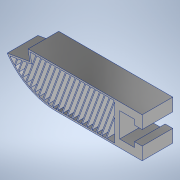
# Autodesk Inventor part: Finray_9_Kerbe_10deg_20deg20inf_PLA
Saved by Autodesk Inventor 2022 (Build 260153000, 153)
## iProperties
Created: 2022-02-28
Part Number: Finray_9_Kerbe_10deg_20deg20inf_PLA
Material: Generic
Document SubType Name: Modeling
Designer: richa
Density: 1 g/cm^3
Appearance: Aluminum - Flat
Author: richa
Autodesk Inventor part; units mm, degrees
ref_plane "YZ Plane" through (0, 0, 0) normal (1, 0, 0) x (0, 1, 0)
ref_plane "XZ Plane" through (0, 0, 0) normal (0, 1, 0) x (-1, 0, 0)
ref_plane "XY Plane" through (0, 0, 0) normal (0, 0, 1) x (1, 0, 0)
sketch "Sketch5" plane through (0, 0, 0) normal (0, 0, 1) x (1, 0, 0)
  line L0 (52.8, -15.6) -> (52.8, -10.6)
  line L1 (52.8, -10.6) -> (49.8, -10.6)
  line L2 (49.8, -10.6) -> (49.8, -12.6)
  line L3 (44, -12.6) -> (44, -3)
  line L4 (49.8, -3) -> (49.8, -5)
  line L5 (49.8, -5) -> (52.8, -5)
  line L6 (52.8, -5) -> (52.8, 0)
  line L7 (52.8, 0) -> (7.8, 0)
  line L8 (44, -3) -> (49.8, -3)
  line L9 (44, -12.6) -> (49.8, -12.6)
  line L10 (52.8, -15.6) -> (7.8, -15.6)
  line L11 (7.8, -15.6) -> (0, -15.6)
  line L12 (0, -15.6) -> (0, 0)
  line L13 (0, 0) -> (7.8, 0)
  point P0 (7.8, 0)
  dimension "d41" = 5.8
  dimension "d48" = 44
  dimension "d50" = 3
  dimension "d63" = 45
  dimension "d71" = 0
  dimension "d87" = 5.6
  dimension "d88" = 9.6
  dimension "d97" = 15.6
  constraints: 28 end point, 8 perpendicular, 4 collinear, 3 parallel, 2 horizontal, 1 vertical
  measures "d41" distance between parallel lines of L2 L3
  measures "d48" distance from line of L3 L12.end
  measures "d50" distance of L4.end L5.end
  measures "d63" distance of L0.start L10.end
  measures "d71" distance from line of L12.end L7
  measures "d87" distance from line of L0.end L5
  measures "d88" distance of L3.start L3.end
  measures "d97" distance of L11.end L12.end
extrude "Extrusion2" add sketch "Sketch5" along normal blind 12
sketch "Sketch8" plane through (0, 0, 0) normal (0, 0, -1) x (-1, 0, 0)
  line L0 (-8.1687, 0) -> (-8.8633, -3.9392)
  line L1 (-7.8, 0) -> (-1.143, 0) construction
  line L2 (0, -5.5021) -> (-8.8633, -3.9392)
  line L3 (-7.8, 0) -> (-8.1687, 0)
  line L4 (0, 0) -> (0, -15.6) projected
  line L5 (-52.8, 0) -> (0, 0) projected
  line L6 (-7.8, 0) -> (0, 0)
  line L7 (0, 0) -> (0, -5.5021)
  dimension "d80" = 100
  dimension "d95" = 4
  dimension "d96" = 9
  constraints: 12 end point, 2 collinear, 2 perpendicular, 1 horizontal, 1 point on line
  measures "d80" angle of L0 L1
  measures "d95" distance of L0.start L0.end
  measures "d96" distance of L2.start L0.end
extrude "Extrusion5" cut sketch "Sketch8" against normal through all
fillet "Fillet2" radius 23 1 edges at (0, -15.6, 6)
shell "Shell1" thickness 0.62 removed faces 1 at (23.9679, -7.5131, 12)
sketch "Sketch13" plane through (0, 0, 12) normal (0, 0, 1) x (1, 0, 0)
  line L0 (19.0404, -15.6) -> (52.8, -15.6) projected
  line L1 (42.0526, -15.6) -> (42.0526, 0)
  line L2 (52.8, 0) -> (8.1687, 0) projected
  line L3 (52.8, 0) -> (8.1687, 0) projected
  line L4 (52.8, -5) -> (52.8, 0) projected
  line L5 (49.8, -5) -> (52.8, -5) projected
  line L6 (49.8, -3) -> (49.8, -5) projected
  line L7 (44, -3) -> (49.8, -3) projected
  line L8 (44, -12.6) -> (44, -3) projected
  line L9 (49.8, -12.6) -> (44, -12.6) projected
  line L10 (49.8, -10.6) -> (49.8, -12.6) projected
  line L11 (52.8, -10.6) -> (49.8, -10.6) projected
  line L12 (52.8, -15.6) -> (52.8, -10.6) projected
  line L13 (42.0526, 0) -> (52.8, 0)
  line L14 (52.8, -5) -> (52.8, 0) projected
  line L15 (52.8, -5) -> (52.8, 0)
  line L16 (52.8, 0) -> (52.8, -5)
  line L17 (44, -12.6) -> (44, -3) projected
  line L18 (44, -3) -> (44, -12.6)
  line L19 (49.8, -12.6) -> (44, -12.6) projected
  line L20 (44, -12.6) -> (49.8, -12.6)
  line L21 (43.38, -13.22) -> (50.42, -13.22) projected
  line L22 (52.8, -10.6) -> (52.8, -15.6)
  line L23 (52.8, -15.6) -> (42.0526, -15.6)
  line L24 (44, -3) -> (49.8, -3) projected
  line L25 (44, -3) -> (49.8, -3)
  line L26 (49.8, -3) -> (49.8, -5)
  line L27 (49.8, -5) -> (52.8, -5)
  line L28 (52.8, -10.6) -> (49.8, -10.6)
  line L29 (49.8, -10.6) -> (49.8, -12.6)
  point P0 (0, 0)
  dimension "d102" = 10.7474
  constraints: 26 end point, 10 collinear, 2 point on line, 2 vertical, 1 parallel
  measures "d102" distance between parallel lines of L4 L1
extrude "Extrusion7" add sketch "Sketch13" against normal blind 12
sketch "Sketch14" plane through (8.9076, -0.62, 0.62) normal (0, 0, 1) x (1, 0, 0)
  line L0 (33.145, -14.36) -> (33.145, 0) projected
  line L1 (33.145, 0) -> (0, 0) projected
  line L2 (0.6739, -3.8221) -> (0, 0) projected
  line L3 (-7.835, -5.3225) -> (0.6739, -3.8221) projected
  arc A0 (-7.835, -5.3225) -> (10.1328, -14.36) centre (10.1328, 8.02) ccw projected
  line L4 (10.1328, -14.36) -> (33.145, -14.36) projected
  point P0 (-8.9076, 0.62)
extrude "Extrusion8" cut sketch "Sketch14" against normal blind 12
sketch "Sketch15" plane through (0, 0, 12) normal (0, 0, 1) x (1, 0, 0)
  line L0 (42.0526, -0.62) -> (8.9076, -0.62) construction
  line L1 (19.0404, -14.98) -> (42.0526, -14.98) projected
  line L2 (43.7528, -0.49) -> (44.1099, -0.62)
  line L3 (44.1099, -0.62) -> (38.836, -15.11)
  line L4 (38.836, -15.11) -> (38.4789, -14.98)
  line L5 (38.4789, -14.98) -> (43.7528, -0.49)
  arc A0 (1.0726, -5.9425) -> (19.0404, -14.98) centre (19.0404, 7.4) ccw projected
  line L6 (42.0526, -0.62) -> (42.0526, -14.98) projected
  line L7 (1.0726, -5.9425) -> (9.5815, -4.4421) projected
  arc A1 (0, -5.5021) -> (19.0404, -15.6) centre (19.0404, 7.4) ccw projected
  line L8 (42.0526, -14.98) -> (19.0404, -14.98) projected
  line L9 (8.9076, -0.62) -> (42.0526, -0.62) projected
  line L10 (40.2999, -0.62) -> (35.0733, -14.98)
  line L11 (39.8955, -0.62) -> (34.6689, -14.98)
  line L12 (32.6799, -0.62) -> (27.4533, -14.98)
  line L13 (32.2755, -0.62) -> (27.0489, -14.98)
  line L14 (28.8699, -0.62) -> (23.6433, -14.98)
  line L15 (28.4655, -0.62) -> (23.2389, -14.98)
  line L16 (25.0599, -0.62) -> (19.8333, -14.98)
  line L17 (24.6555, -0.62) -> (19.4289, -14.98)
  line L18 (21.1404, -0.62) -> (15.9898, -14.7711)
  line L19 (17.3304, -0.62) -> (12.4634, -13.9918)
  line L20 (16.926, -0.62) -> (12.1009, -13.8769)
  line L21 (13.5204, -0.62) -> (9.135, -12.6686)
  line L22 (13.116, -0.62) -> (8.7934, -12.4963)
  line L23 (7.8054, -0.62) -> (4.5246, -9.6339)
  line L24 (7.401, -0.62) -> (4.2173, -9.3672)
  line L25 (20.736, -0.62) -> (15.6059, -14.7149)
  line L26 (36.4899, -0.62) -> (31.2633, -14.98)
  line L27 (36.0855, -0.62) -> (30.8589, -14.98)
  line L28 (41.8005, -0.62) -> (36.5739, -14.98)
  line L29 (42.2049, -0.62) -> (36.9783, -14.98)
  line L30 (37.9905, -0.62) -> (32.7639, -14.98)
  line L31 (38.3949, -0.62) -> (33.1683, -14.98)
  line L32 (34.1805, -0.62) -> (28.9539, -14.98)
  line L33 (34.5849, -0.62) -> (29.3583, -14.98)
  line L34 (30.3705, -0.62) -> (25.1439, -14.98)
  line L35 (30.7749, -0.62) -> (25.5483, -14.98)
  line L36 (26.5605, -0.62) -> (21.3339, -14.98)
  line L37 (26.9649, -0.62) -> (21.7383, -14.98)
  line L38 (22.7505, -0.62) -> (17.5422, -14.9298)
  line L39 (23.1549, -0.62) -> (17.9382, -14.9528)
  line L40 (18.831, -0.62) -> (13.8283, -14.3646)
  line L41 (19.2354, -0.62) -> (14.2014, -14.4506)
  line L42 (15.021, -0.62) -> (10.4225, -13.2542)
  line L43 (15.4254, -0.62) -> (10.7747, -13.3977)
  line L44 (11.211, -0.62) -> (7.2145, -11.6003)
  line L45 (11.6154, -0.62) -> (7.5453, -11.8023)
  line L46 (9.7104, -0.62) -> (6.0075, -10.7936)
  line L47 (9.306, -0.62) -> (5.688, -10.5604)
  line L48 (5.496, -0.62) -> (2.8075, -8.0064)
  line L49 (5.9004, -0.62) -> (3.1014, -8.3102)
  line L50 (9.5815, -4.4421) -> (8.9076, -0.62) construction
  line L51 (8.9076, -0.62) -> (-0.1181, -0.62) construction
  point P0 (0, 0)
  point P1 (38.4789, -14.98)
  point P2 (6.197, -5.0389)
  point P3 (5.7649, -5.1151)
  point P4 (38.8833, -14.98)
  point P5 (38.4789, -14.98)
  point P6 (35.0733, -14.98)
  point P7 (30.8589, -14.98)
  point P8 (31.2633, -14.98)
  point P9 (27.0489, -14.98)
  point P10 (27.4533, -14.98)
  point P11 (23.2389, -14.98)
  point P12 (23.6433, -14.98)
  point P13 (19.4289, -14.98)
  point P14 (19.8333, -14.98)
  point P15 (8.2327, -4.68)
  point P16 (7.8005, -4.7562)
  point P17 (3.7292, -5.4741)
  point P18 (4.1614, -5.3979)
  point P19 (36.9783, -14.98)
  point P20 (42.0526, -1.0384)
  point P21 (33.1683, -14.98)
  point P22 (32.7639, -14.98)
  point P23 (29.3583, -14.98)
  point P24 (28.9539, -14.98)
  point P25 (25.5483, -14.98)
  point P26 (25.1439, -14.98)
  point P27 (21.7383, -14.98)
  point P28 (21.3339, -14.98)
  dimension "d105" = 0.38
  dimension "d130" = 110
  dimension "d132" = 110
  dimension "d133" = 0.38
  dimension "d135" = 0.38
  dimension "d136" = 0.38
  dimension "d137" = 0.38
  dimension "d138" = 0.38
  dimension "d139" = 0.38
  dimension "d140" = 0.38
  dimension "d141" = 0.38
  dimension "d142" = 3.81
  dimension "d143" = 0.38
  dimension "d144" = 3.81
  dimension "d145" = 3.81
  dimension "d146" = 3.81
  dimension "d147" = 3.81
  dimension "d152" = 110
  dimension "d153" = 0.38
  dimension "d154" = 0.38
  dimension "d155" = 0.38
  dimension "d156" = 0.38
  dimension "d157" = 0.38
  dimension "d158" = 0.38
  dimension "d159" = 0.38
  dimension "d160" = 0.38
  dimension "d161" = 0.38
  dimension "d162" = 0.38
  dimension "d163" = 1.905
  dimension "d164" = 1.905
  dimension "d165" = 1.905
  dimension "d166" = 1.905
  dimension "d167" = 1.905
  dimension "d168" = 1.905
  dimension "d169" = 1.905
  dimension "d170" = 1.905
  dimension "d171" = 3.9195
  dimension "d172" = 3.81
  dimension "d173" = 3.81
  dimension "d175" = 1.905
  dimension "d180" = 0.38
  dimension "d182" = 1.905
  dimension "d183" = 1.905
  dimension "d184" = 1.905
  constraints: 90 end point, 40 parallel, 16 point on line, 1 horizontal, 1 perpendicular, 82 other
  measures "d105" distance between parallel lines of L3 L5
  measures "d130" angle of L0 L3
  measures "d132" angle of L0 L10
  measures "d133" distance between parallel lines of L10 L11
  measures "d135" distance between parallel lines of L13 L12
  measures "d136" distance between parallel lines of L15 L14
  measures "d137" distance between parallel lines of L17 L16
  measures "d138" distance between parallel lines of L25 L18
  measures "d139" distance between parallel lines of L20 L19
  measures "d140" distance between parallel lines of L22 L21
  measures "d141" distance between parallel lines of L24 L23
  measures "d142" distance of L4.end L11.end
  measures "d143" distance between parallel lines of L26 L27
  measures "d144" distance of L11.end L27.end
  measures "d145" distance of L27.end L13.end
  measures "d146" distance of L15.end L13.end
  measures "d147" distance of L15.end L17.end
  measures "d152" angle of L0 L12
  measures "d153" distance between parallel lines of L29 L28
  measures "d154" distance between parallel lines of L31 L30
  measures "d155" distance between parallel lines of L32 L33
  measures "d156" distance between parallel lines of L34 L35
  measures "d157" distance between parallel lines of L36 L37
  measures "d158" distance between parallel lines of L38 L39
  measures "d159" distance between parallel lines of L40 L41
  measures "d160" distance between parallel lines of L42 L43
  measures "d161" distance between parallel lines of L44 L45
  measures "d162" distance between parallel lines of L47 L46
  measures "d163" distance of L28.end L4.end
  measures "d164" distance of L30.end L11.end
  measures "d165" distance of L32.end L27.end
  measures "d166" distance of L13.end L34.end
  measures "d167" distance of L36.end L15.end
  measures "d168" distance of L38.start L17.start
  measures "d169" distance of L40.start L25.start
  measures "d170" distance of L42.start L20.start
  measures "d171" distance of L25.start L17.start
  measures "d172" distance of L42.start L40.start
  measures "d173" distance of L44.start L42.start
  measures "d175" distance of L22.start L42.start
  measures "d180" distance between parallel lines of L49 L48
  measures "d182" distance of L47.start L44.start
  measures "d183" distance of L47.start L24.start
  measures "d184" distance of L24.start L48.start
extrude "Extrusion9" add sketch "Sketch15" against normal blind 12 contours L17 L9 L16 L1 | A0 L38 L9 L39 | L36 L9 L37 L1 | A0 L25 L9 L18 | L15 L9 L14 L1 | A0 L40 L9 L41 | L34 L9 L35 L1 | A0 L20 L9 L19 | L13 L9 L12 L1 | A0 L42 L9 L43 | L32 L9 L33 L1 | A0 L22 L9 L21 | L27 L9 L26 L1 | A0 L44 L9 L45 | L30 L9 L31 L1 | A0 L47 L7 L46 | L11 L9 L10 L1 | A0 L24 L7 L23 | L28 L9 L6 L29 L1 | A0 L48 L7 L49 | L5 L6 L3 L1 | L5 L2 L3 L6
equation "\"l1\" = 8"
equation "\"d1\" = 0.38"
body "Solid2"
